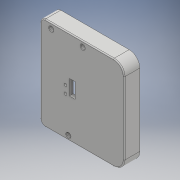
# Autodesk Inventor part: back
Saved by Autodesk Inventor 2017 (Build 210142000, 142)
## iProperties
Created: 2017-07-30
Part Number: back
Material: Generic
Document SubType Name: Modeling
Designer: Käyttäjä
Density: 1 g/cm^3
Appearance: Default
Author: Käyttäjä
Autodesk Inventor part; units mm, degrees
ref_plane "YZ Plane" through (0, 0, 0) normal (1, 0, 0) x (0, 1, 0)
ref_plane "XZ Plane" through (0, 0, 0) normal (0, 1, 0) x (-1, 0, 0)
ref_plane "XY Plane" through (0, 0, 0) normal (0, 0, 1) x (1, 0, 0)
sketch "Sketch1" plane through (0, 0, 0) normal (0, 1, 0) x (-1, 0, 0)
  line L0 (10, 0) -> (82, 0)
  line L1 (86, -4) -> (86, -92)
  line L2 (82, -96) -> (10, -96)
  line L3 (0, -86) -> (0, -10)
  arc A0 (10, 0) -> (0, -10) centre (10, -10) ccw
  arc A1 (0, -86) -> (10, -96) centre (10, -86) ccw
  arc A2 (86, -4) -> (82, 0) centre (82, -4) ccw
  arc A3 (82, -96) -> (86, -92) centre (82, -92) ccw
  line L4 (87.2, -92) -> (87.2, -4)
  arc A4 (87.2, -4) -> (82, 1.2) centre (82, -4) ccw
  line L5 (82, 1.2) -> (10, 1.2)
  arc A5 (10, 1.2) -> (-1.2, -10) centre (10, -10) ccw
  line L6 (-1.2, -10) -> (-1.2, -86)
  arc A6 (-1.2, -86) -> (10, -97.2) centre (10, -86) ccw
  line L7 (10, -97.2) -> (82, -97.2)
  arc A7 (82, -97.2) -> (87.2, -92) centre (82, -92) ccw
  point P0 (0, 0)
  point P1 (86, 0)
  point P2 (0, -96)
  dimension "d0" = 96
  dimension "d1" = 86
  dimension "d2" = 10
  dimension "d3" = 4
  dimension "d4" = 1.2
  constraints: 16 end point, 16 point on circle, 8 centre point, 8 tangent, 6 point on line, 4 parallel, 2 equal radius, 2 perpendicular, 1 horizontal, 7 other
  measures "d0" distance of point (0, -96) point (0, 0)
  measures "d1" distance of point (0, 0) point (86, 0)
  measures "d2" radius of A0
  measures "d3" radius of A2
  measures "d4" distance between parallel lines of L1 L4
extrude "walls" add sketch "Sketch1" along normal blind 15.5
sketch "Sketch2" plane through (0, 0, 0) normal (0, -1, 0) x (1, 0, 0)
  arc A0 (-82, 0) -> (-86, -4) centre (-82, -4) ccw projected
  line L0 (-82, 0) -> (-10, 0) projected
  arc A1 (0, -10) -> (-10, 0) centre (-10, -10) ccw projected
  line L1 (0, -10) -> (0, -86) projected
  arc A2 (-10, -96) -> (0, -86) centre (-10, -86) ccw projected
  line L2 (-10, -96) -> (-82, -96) projected
  arc A3 (-86, -92) -> (-82, -96) centre (-82, -92) ccw projected
  line L3 (-86, -92) -> (-86, -4) projected
  line L4 (-87.2, -92) -> (-87.2, -4) projected
  arc A4 (-87.2, -92) -> (-82, -97.2) centre (-82, -92) ccw projected
  line L5 (-10, -97.2) -> (-82, -97.2) projected
  arc A5 (-10, -97.2) -> (1.2, -86) centre (-10, -86) ccw projected
  line L6 (1.2, -10) -> (1.2, -86) projected
  arc A6 (1.2, -10) -> (-10, 1.2) centre (-10, -10) ccw projected
  line L7 (-82, 1.2) -> (-10, 1.2) projected
  arc A7 (-82, 1.2) -> (-87.2, -4) centre (-82, -4) ccw projected
  point P0 (0, 0)
extrude "back" add sketch "Sketch2" along normal blind 1 contours L0 A1 L1 A2 L2 A3 L3 A0 | L4 A7 L7 A6 L6 A5 L5 A4
sketch "Sketch3" plane through (-87.2, 15.5, -92) normal (-1, 0, 0) x (0, 0, 1)
  line L0 (0, -15.5) -> (88, -15.5) projected
  line L1 (92, -15.5) -> (92, 0) projected
  circle A0 centre (88, -5) radius 2
  line L2 (-4, -15.5) -> (-4, 0) projected
  circle A1 centre (0, -5) radius 2
  dimension "d9" = 4
  dimension "d10" = 4
  dimension "d11" = 10.5
  dimension "d12" = 4
  constraints: 2 centre point, 1 equal radius, 1 horizontal alignment
  measures "d9" distance from line of L1 A0.centre
  measures "d10" distance from line of A1.centre L2
  measures "d11" distance from line of L0 A0.centre
  measures "d12" diameter of A0
extrude "string holes" cut sketch "Sketch3" against normal up to next
sketch "Sketch5" plane through (0, 0, 0) normal (0, 1, 0) x (1, 0, 0)
  circle A0 centre (-75.5, 4.5) radius 2.75
  circle A1 centre (-57.5, 92.5) radius 2.75
  line L0 (0, 86) -> (0, 10) projected
  line L1 (-82, 96) -> (-10, 96) projected
  circle A2 centre (-42.5, 4.5) radius 2.75
  point P0 (0, 0)
  dimension "d19" = 5.5
  dimension "d21" = 57.5
  dimension "d22" = 3.5
  dimension "d23" = 91.5
  dimension "d24" = 75.5
  dimension "d25" = 42.5
  constraints: 3 centre point, 2 equal radius, 1 horizontal alignment
  measures "d19" diameter of A0
  measures "d21" distance from line of L0 A1.centre
  measures "d22" distance from line of L1 A1.centre
  measures "d23" distance from line of A0.centre L1
  measures "d24" distance from line of L0 A0.centre
  measures "d25" distance from line of A2.centre L0
extrude "PCB pillars" add sketch "Sketch5" along normal blind 10.5
sketch "Sketch6" plane through (-10, 15.5, -97.2) normal (0, 0, -1) x (-1, 0, 0)
  line L0 (44, 0) -> (29, 0)
  line L1 (29, 0) -> (29, -8.5)
  line L2 (29, -8.5) -> (44, -8.5)
  line L3 (44, -8.5) -> (44, 0)
  line L4 (-10, -15.5) -> (-10, 0) projected
  line L5 (0, 0) -> (72, 0) projected
  line L6 (0, -15.5) -> (72, -15.5) projected
  dimension "d28" = 39
  dimension "d29" = 54
  dimension "d30" = 7
  constraints: 8 end point, 2 parallel, 1 horizontal, 1 perpendicular, 1 point on line
  measures "d28" distance between parallel lines of L4 L1
  measures "d29" distance between parallel lines of L4 L3
  measures "d30" distance between parallel lines of L2 L6
sketch "Sketch7" plane through (-75.5, 10.5, -4.5) normal (0, 1, 0) x (1, 0, 0)
  circle A0 centre (0, 0) radius 2.75 projected
  circle A1 centre (0, 0) radius 1.75
  circle A2 centre (33, 0) radius 2.75 projected
  circle A3 centre (18, 88) radius 2.75 projected
  circle A4 centre (33, 0) radius 1.75
  circle A5 centre (18, 88) radius 1.75
  point P0 (75.5, -4.5)
  dimension "d31" = 3.5
  constraints: 3 centre point, 3 coincident, 2 equal radius
  measures "d31" diameter of A1
sketch "Sketch8" plane through (-87.2, 15.5, -92) normal (-1, 0, 0) x (0, 0, 1)
  line L0 (-4, -15.5) -> (-4, 0) projected
  line L1 (92, -15.5) -> (92, 0) projected
  line L2 (88, 0) -> (0, 0) projected
  line L3 (39, 0) -> (49, 0)
  line L4 (49, 0) -> (49, -10.1)
  line L5 (49, -10.1) -> (39, -10.1)
  line L6 (39, -10.1) -> (39, 0)
  line L7 (0, -15.5) -> (88, -15.5) projected
  point P0 (44, -15.5)
  point P1 (44, -10.1)
  dimension "d34" = 5.4
  dimension "d35" = 10
  constraints: 8 end point, 2 midpoint, 2 parallel, 1 horizontal, 1 perpendicular, 1 point on line, 1 vertical alignment
  measures "d34" distance between parallel lines of L7 L5
  measures "d35" distance of L4.end L5.end
extrude "Extrusion5" cut sketch "Sketch8" against normal blind 9.5
extrude "Extrusion6" cut sketch "Sketch7" against normal through all contours A1 | A4 | A5
sketch "Sketch9" plane through (0, 0, 0) normal (0, 1, 0) x (1, 0, 0)
  circle A0 centre (-75.5, 4.5) radius 1.75 projected
  circle A1 centre (-42.5, 4.5) radius 1.75 projected
  circle A2 centre (-57.5, 92.5) radius 1.75 projected
  circle A3 centre (-57.5, 92.5) radius 2.75 projected
  circle A4 centre (-75.5, 4.5) radius 2.75 projected
  circle A5 centre (-42.5, 4.5) radius 2.75 projected
  arc A6 (-86, 4) -> (-82, 0) centre (-82, 4) ccw projected
  line L0 (-82, 0) -> (-10, 0) projected
  arc A7 (-10, 0) -> (0, 10) centre (-10, 10) ccw projected
  line L1 (0, 10) -> (0, 86) projected
  arc A8 (0, 86) -> (-10, 96) centre (-10, 86) ccw projected
  line L2 (-10, 96) -> (-82, 96) projected
  arc A9 (-82, 96) -> (-86, 92) centre (-82, 92) ccw projected
  line L3 (-86, 92) -> (-86, 4) projected
  circle A10 centre (-42.5, 4.5) radius 2.75 projected
  circle A11 centre (-57.5, 92.5) radius 2.75 projected
  circle A12 centre (-75.5, 4.5) radius 5.7
  line L4 (-10, 0) -> (-82, 0) projected
  circle A13 centre (-42.5, 4.5) radius 5.7
  circle A14 centre (-57.5, 92.5) radius 4.7
  line L5 (-82, 96) -> (-10, 96) projected
  line L6 (-10, -1.2) -> (-82, -1.2) projected
  line L7 (-82, 97.2) -> (-10, 97.2) projected
  point P0 (0, 0)
  constraints: 3 centre point, 3 coincident, 2 tangent, 1 equal radius
extrude "Extrusion7" add sketch "Sketch9" along normal blind 3 contours A12 L0 | L0 A12 | A14 L2 | L2 A14 | A13 L0 | L0 A13
extrude "Extrusion8" cut sketch "Sketch6" against normal blind 3
sketch "Sketch11" plane through (0, 0, 0) normal (0, 1, 0) x (1, 0, 0)
  arc A0 (-86, 4) -> (-82, 0) centre (-82, 4) ccw projected
  line L0 (-39.0014, 0) -> (-10, 0) projected
  arc A1 (-72.0014, 0) -> (-78.9986, 0) centre (-75.5, 4.5) ccw projected
  arc A2 (-39.0014, 0) -> (-45.9986, 0) centre (-42.5, 4.5) ccw projected
  arc A3 (-10, 0) -> (0, 10) centre (-10, 10) ccw projected
  line L1 (0, 10) -> (0, 86) projected
  arc A4 (0, 86) -> (-10, 96) centre (-10, 86) ccw projected
  line L2 (-10, 96) -> (-54.3631, 96) projected
  arc A5 (-60.6369, 96) -> (-54.3631, 96) centre (-57.5, 92.5) ccw projected
  arc A6 (-82, 96) -> (-86, 92) centre (-82, 92) ccw projected
  line L3 (-86, 92) -> (-86, 4) projected
  line L4 (-40, 0) -> (-40, 96)
  line L5 (-10, 96) -> (-54.3631, 96) projected
  line L6 (-82, 0) -> (-78.9986, 0) projected
  line L7 (-40, 9.6225) -> (0, 9.6225)
  line L8 (-60.6369, 96) -> (-82, 96) projected
  line L9 (-72.0014, 0) -> (-45.9986, 0) projected
  point P0 (0, 0)
  point P1 (-57.5, 96)
  dimension "d45" = 40
  constraints: 4 end point, 3 point on line, 2 perpendicular, 1 point on circle, 1 other
  measures "d45" distance between parallel lines of L4 L1
fillet "Fillet3" radius 1 2 edges at (-86.6, 5.4, -53) (-86.6, 5.4, -43)
sketch "Sketch12" plane through (-57.5, 10.5, -92.5) normal (0, 1, 0) x (1, 0, 0)
  circle A0 centre (0, 0) radius 1.75 projected
  circle A1 centre (0, 0) radius 2.75 projected
  circle A2 centre (0, 0) radius 2.75 projected
  line L0 (-1.8, 2.0791) -> (-1.8, -2.0791)
  point P0 (57.5, -92.5)
  dimension "d57" = 1.8
  constraints: 4 point on circle, 2 end point, 1 vertical
  measures "d57" distance from line of L0 A0.centre
extrude "room for esp" cut sketch "Sketch12" against normal blind 2.5 contours L0 A1 picked at (-1.9501, -0.5269)
fillet "Fillet4" radius 2 3 edges at (-78.25, 3, -4.5) (-45.25, 3, -4.5) (-60.25, 3, -92.5)
extrude "Extrusion13" [suppressed]
sketch "Sketch13" plane through (0, -1, 0) normal (0, -1, 0) x (1, 0, 0)
  circle A0 centre (-42.5, -4.5) radius 1.75 projected
  circle A1 centre (-75.5, -4.5) radius 1.75 projected
  circle A2 centre (-57.5, -92.5) radius 1.75 projected
  line L0 (-87.2, -4) -> (-87.2, -92) projected
  arc A3 (-87.2, -92) -> (-82, -97.2) centre (-82, -92) ccw projected
  line L1 (-82, -97.2) -> (-10, -97.2) projected
  arc A4 (-10, -97.2) -> (1.2, -86) centre (-10, -86) ccw projected
  line L2 (1.2, -86) -> (1.2, -10) projected
  arc A5 (1.2, -10) -> (-10, 1.2) centre (-10, -10) ccw projected
  line L3 (-10, 1.2) -> (-82, 1.2) projected
  arc A6 (-82, 1.2) -> (-87.2, -4) centre (-82, -4) ccw projected
  circle A7 centre (-57.5, -92.5) radius 2.25
  circle A8 centre (-42.5, -4.5) radius 2.25
  circle A9 centre (-75.5, -4.5) radius 2.25
  point P0 (0, 0)
  dimension "d77" = 4.5
  dimension "d78" = 4.5
  dimension "d79" = 4.5
  constraints: 3 centre point, 3 coincident
  measures "d77" diameter of A7
  measures "d78" diameter of A9
  measures "d79" diameter of A8
extrude "inser holes" cut sketch "Sketch13" against normal blind 5 contours A7 | A8 | A9
fillet "Fillet6" radius 0.5 3 edges at (-59.75, -1, -92.5) (-77.75, -1, -4.5) (-44.75, -1, -4.5)
fillet "Fillet7" radius 1 8 edges at (-2.0804, -1, -93.9196) (1.2, -1, -48) (-2.0804, -1, -2.0804) (-46, -1, 1.2) (-85.677, -1, -0.323) (-87.2, -1, -48) (-85.677, -1, -95.677) (-46, -1, -97.2)
chamfer "Chamfer6" [suppressed]
chamfer "Chamfer7" [suppressed]
fillet "Fillet8" [suppressed]
fillet "Fillet9" [suppressed]
fillet "Fillet10" [suppressed]
chamfer "Chamfer8" distance 0.5 angle 45 1 edges at (-59.75, 4, -92.5) measured on face at (-59.65, 4, -92.5)
chamfer "Chamfer9" distance 0.5 angle 45 1 edges at (-77.75, 4, -4.5) measured on face at (-77.65, 4, -4.5)
chamfer "Chamfer10" distance 0.5 angle 45 1 edges at (-44.75, 4, -4.5) measured on face at (-44.65, 4, -4.5)
fillet "Fillet11" radius 0.5 5 edges at (-87.2, 5.6929, -52.7071) (-87.2, 5.4, -48) (-87.2, 5.6929, -43.2929) (-87.2, 10.95, -43) (-87.2, 10.95, -53)
sketch "Sketch14" plane through (0, 0, 0) normal (0, 1, 0) x (1, 0, 0)
  arc A0 (-86.7, 43) -> (-87.2, 42.5) centre (-86.7, 42.5) ccw projected
  line L0 (-87.2, 42.5) -> (-87.2, 4) projected
  arc A1 (-87.2, 4) -> (-82, -1.2) centre (-82, 4) ccw projected
  line L1 (-82, -1.2) -> (-10, -1.2) projected
  arc A2 (-10, -1.2) -> (1.2, 10) centre (-10, 10) ccw projected
  line L2 (1.2, 10) -> (1.2, 86) projected
  arc A3 (1.2, 86) -> (-10, 97.2) centre (-10, 86) ccw projected
  line L3 (-10, 97.2) -> (-39, 97.2) projected
  line L4 (-39, 97.2) -> (-39, 96) projected
  line L5 (-39, 96) -> (-10, 96) projected
  arc A4 (0, 86) -> (-10, 96) centre (-10, 86) ccw projected
  line L6 (0, 86) -> (0, 10) projected
  arc A5 (-10, 0) -> (0, 10) centre (-10, 10) ccw projected
  line L7 (-10, 0) -> (-82, 0) projected
  arc A6 (-86, 4) -> (-82, 0) centre (-82, 4) ccw projected
  line L8 (-86, 4) -> (-86, 43) projected
  line L9 (-86, 43) -> (-86.7, 43) projected
  line L10 (-56.5, 40) -> (-50.5, 40)
  line L11 (-50.5, 40) -> (-50.5, 56)
  line L12 (-50.5, 56) -> (-56.5, 56)
  line L13 (-56.5, 56) -> (-56.5, 40)
  line L14 (0, 86) -> (0, 10) projected
  point P0 (0, 0)
  point P1 (-56.5, 48)
  point P2 (0, 48)
  dimension "d103" = 50.5
  dimension "d104" = 56.5
  dimension "d105" = 16
  constraints: 8 end point, 2 midpoint, 2 parallel, 1 horizontal, 1 horizontal alignment, 1 perpendicular
  measures "d103" distance between parallel lines of L6 L11
  measures "d104" distance between parallel lines of L6 L13
  measures "d105" distance of L12.end L10.start
extrude "Extrusion15" cut sketch "Sketch14" against normal blind 5 contours L13 L12 L11 L10
fillet "Fillet12" [suppressed]
fillet "Fillet13" radius 0.5 6 edges at (-86.8, 10.5005, -94) (-87.2, 9.0858, -90.5858) (-87.2, 11.9142, -90.5858) (-87.2, 10.5, -6) (-86.9774, 9.1829, -2.4949) (-86.9773, 11.8167, -2.4946)
sketch "Sketch16" plane through (0, 0, 0) normal (0, 1, 0) x (1, 0, 0)
  line L0 (-50.5, 56) -> (-50.5, 40) projected
  line L1 (-50.5, 40) -> (-56.5, 40) projected
  line L2 (-56.5, 40) -> (-56.5, 56) projected
  line L3 (-56.5, 56) -> (-50.5, 56) projected
  arc A0 (-39.0014, 0) -> (-45.9986, 0) centre (-42.5, 4.5) ccw projected
  line L4 (-39.0014, 0) -> (-10, 0) projected
  arc A1 (-10, 0) -> (0, 10) centre (-10, 10) ccw projected
  line L5 (0, 10) -> (0, 86) projected
  arc A2 (0, 86) -> (-10, 96) centre (-10, 86) ccw projected
  line L6 (-10, 96) -> (-54.3631, 96) projected
  arc A3 (-60.6369, 96) -> (-54.3631, 96) centre (-57.5, 92.5) ccw projected
  line L7 (-60.6369, 96) -> (-82, 96) projected
  arc A4 (-82, 96) -> (-86, 92) centre (-82, 92) ccw projected
  line L8 (-86, 92) -> (-86, 4) projected
  arc A5 (-86, 4) -> (-82, 0) centre (-82, 4) ccw projected
  line L9 (-82, 0) -> (-78.9986, 0) projected
  arc A6 (-72.0014, 0) -> (-78.9986, 0) centre (-75.5, 4.5) ccw projected
  line L10 (-72.0014, 0) -> (-45.9986, 0) projected
  line L11 (-58.5, 58) -> (-58.5, 38)
  line L12 (-58.5, 38) -> (-48.5, 38)
  line L13 (-48.5, 38) -> (-48.5, 58)
  line L14 (-48.5, 58) -> (-58.5, 58)
  point P0 (0, 0)
  dimension "d110" = 2
  constraints: 8 end point, 3 other
  measures "d110" distance between parallel lines of L2 L11
extrude "connector" add sketch "Sketch16" along normal blind 3 contours L14 L13 L12 L11
sketch "Sketch17" plane through (0, 0, 0) normal (0, 1, 0) x (1, 0, 0)
  circle A0 centre (-60.5, 48) radius 1.5
  circle A1 centre (-60.5, 56) radius 1.5
  line L0 (0, 86) -> (0, 10) projected
  line L1 (-82, 96) -> (-54, 96) projected
  point P0 (0, 0)
  dimension "d113" = 3
  dimension "d114" = 60.5
  dimension "d115" = 40
  dimension "d116" = 48
  constraints: 2 centre point, 1 equal radius, 1 vertical alignment
  measures "d113" diameter of A1
  measures "d114" distance from line of A0.centre L0
  measures "d115" distance from line of A1.centre L1
  measures "d116" distance from line of L1 A0.centre
extrude "Extrusion17" cut sketch "Sketch17" against normal through all
sketch "Sketch18" plane through (0, 0, 0) normal (0, 1, 0) x (1, 0, 0)
  circle A0 centre (-60.5, 48) radius 1.5 projected
  circle A1 centre (-60.5, 56) radius 1.5 projected
  circle A2 centre (-60.5, 48) radius 2.5
  circle A3 centre (-60.5, 56) radius 2.5
  point P0 (0, 0)
  dimension "d119" = 5
  dimension "d120" = 5
  constraints: 2 centre point, 2 coincident
  measures "d119" diameter of A2
  measures "d120" diameter of A3
extrude "Extrusion18" add sketch "Sketch18" along normal blind 3
sketch "Sketch19" plane through (0, 0, 0) normal (0, 1, 0) x (1, 0, 0)
  arc A0 (-39.0014, 0) -> (-45.9986, 0) centre (-42.5, 4.5) ccw projected
  line L0 (-39.0014, 0) -> (-10, 0) projected
  arc A1 (-10, 0) -> (0, 10) centre (-10, 10) ccw projected
  line L1 (0, 10) -> (0, 86) projected
  arc A2 (0, 86) -> (-10, 96) centre (-10, 86) ccw projected
  line L2 (-10, 96) -> (-54.3631, 96) projected
  arc A3 (-60.6369, 96) -> (-54.3631, 96) centre (-57.5, 92.5) ccw projected
  line L3 (-60.6369, 96) -> (-82, 96) projected
  arc A4 (-82, 96) -> (-86, 92) centre (-82, 92) ccw projected
  line L4 (-86, 92) -> (-86, 4) projected
  arc A5 (-86, 4) -> (-82, 0) centre (-82, 4) ccw projected
  line L5 (-82, 0) -> (-78.9986, 0) projected
  arc A6 (-72.0014, 0) -> (-78.9986, 0) centre (-75.5, 4.5) ccw projected
  line L6 (-72.0014, 0) -> (-45.9986, 0) projected
  arc A7 (-58.5, 49.5) -> (-58.5, 46.5) centre (-60.5, 48) ccw projected
  line L7 (-58.5, 49.5) -> (-58.5, 54.5) projected
  arc A8 (-58.5, 57.5) -> (-58.5, 54.5) centre (-60.5, 56) ccw projected
  line L8 (-58.5, 57.5) -> (-58.5, 58) projected
  line L9 (-58.5, 58) -> (-48.5, 58) projected
  line L10 (-48.5, 58) -> (-48.5, 38) projected
  line L11 (-48.5, 38) -> (-58.5, 38) projected
  line L12 (-58.5, 38) -> (-58.5, 46.5) projected
  arc A9 (-10, 1.5) -> (-1.5, 10) centre (-10, 10) ccw
  arc A10 (-1.5, 86) -> (-10, 94.5) centre (-10, 86) ccw
  line L13 (-10, 1.5) -> (-10, 0)
  line L14 (-1.5, 10) -> (0, 10)
  line L15 (-10, 94.5) -> (-10, 96)
  line L16 (-1.5, 86) -> (0, 86)
  line L17 (0, 86) -> (0, 10) projected
  line L18 (0, 43) -> (-1.5, 43)
  line L19 (-1.5, 43) -> (-1.5, 53)
  line L20 (-1.5, 53) -> (0, 53)
  line L21 (0, 53) -> (0, 43)
  line L22 (1.2, 10) -> (1.2, 86) projected
  point P0 (0, 0)
  point P1 (1.2, 48)
  point P2 (-1.5, 48)
  dimension "d123" = 1.5
  dimension "d124" = 1.5
  dimension "d125" = 1.5
  dimension "d126" = 10
  constraints: 16 end point, 4 point on circle, 3 perpendicular, 2 centre point, 2 coincident, 2 horizontal, 2 midpoint, 2 parallel, 1 horizontal alignment, 1 point on line, 1 vertical
  measures "d123" radial gap between concentric circles of A10 A2
  measures "d124" radial gap between concentric circles of A9 A1
  measures "d125" distance of L18.start L18.end
  measures "d126" distance of L18.end L19.end
extrude "Extrusion19" add sketch "Sketch19" along normal up to surface (10.5 mm away) contours L13 A9 L14 A1 | L18 L19 L20 L1 | L16 A10 L15 A2
fillet "Fillet14" radius 2 9 edges at (-32.1816, 0, -96) (0, 0, -69.5) (-24.5007, 0, 0) (-59, 0, 0) (-80.4993, 0, 0) (-86, 0, -48) (-84.8284, 0, -94.8284) (-71.3184, 0, -96) (-84.8284, 0, -1.1716)
body "Solid1"
